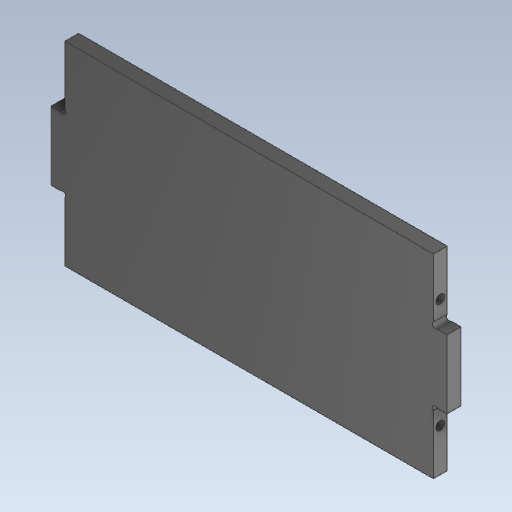
# Autodesk Inventor part: Cockpit_back_frame
Saved by Autodesk Inventor 2020.4 (Build 244396000, 396)
## iProperties
Created: 2022-01-20
Part Number: Cockpit_back_frame
Material: アセタール樹脂、黒
Document SubType Name: Modeling
Designer: Masato Kubotera
Density: 1.425 g/cm^3
Appearance: 滑らか - 黒
Author: Masato Kubotera
Autodesk Inventor part; units mm, degrees
ref_plane "XZ Plane" through (0, 0, 0) normal (0, 1, 0) x (-1, 0, 0)
ref_plane "XY Plane" through (0, 0, 0) normal (0, 0, 1) x (1, 0, 0)
derived "Cockpit_side_frame.ipt"
sketch "スケッチ1" plane through (0, 0, 0) normal (0, 1, 0) x (-1, 0, 0)
  line L0 (-60, 36.75) -> (60, 36.75) construction
  line L1 (60, 36.75) -> (60, -36.75) construction
  line L2 (60, -36.75) -> (-60, -36.75) construction
  line L3 (-60, -36.75) -> (-60, 36.75) construction
  line L4 (-60, 36.75) -> (60, -36.75) construction
  line L5 (60, 36.75) -> (-60, -36.75) construction
  line L6 (-52.5, 6.75) -> (52.5, 6.75) construction
  line L7 (52.5, 6.75) -> (52.5, 1.75) construction
  line L8 (52.5, 1.75) -> (-52.5, 1.75) construction
  line L9 (-52.5, 1.75) -> (-52.5, 6.75) construction
  line L10 (-52.5, 6.75) -> (52.5, 1.75) construction
  line L11 (52.5, 6.75) -> (-52.5, 1.75) construction
  line L12 (0, 36.75) -> (0, -36.75) construction
  line L13 (-57.5, 34.25) -> (-52.5, 34.25) construction
  line L14 (-52.5, 34.25) -> (-52.5, -34.25) construction
  line L15 (-52.5, -34.25) -> (-57.5, -34.25) construction
  line L16 (-57.5, -34.25) -> (-57.5, 34.25) construction
  line L17 (-57.5, 34.25) -> (-52.5, -34.25) construction
  line L18 (-52.5, 34.25) -> (-57.5, -34.25) construction
  line L19 (-55, 36.75) -> (-60, 31.75)
  line L20 (-60, 0) -> (60, 0) construction
  line L21 (-46.5, 41.75) -> (32.5, 41.75) construction
  line L22 (32.5, 41.75) -> (32.5, 11.75) construction
  line L23 (32.5, 11.75) -> (-46.5, 11.75) construction
  line L24 (-46.5, 11.75) -> (-46.5, 41.75) construction
  line L25 (-46.5, 41.75) -> (32.5, 11.75) construction
  line L26 (32.5, 41.75) -> (-46.5, 11.75) construction
  line L27 (-55, -36.75) -> (-60, -31.75)
  line L28 (-60, 31.75) -> (-60, -31.75)
  line L29 (55, -36.75) -> (60, -31.75)
  line L30 (-52.5, -29.25) -> (52.5, -29.25) construction
  line L31 (52.5, -29.25) -> (52.5, -34.25) construction
  line L32 (52.5, -34.25) -> (-52.5, -34.25) construction
  line L33 (-52.5, -34.25) -> (-52.5, -29.25) construction
  line L34 (-52.5, -29.25) -> (52.5, -34.25) construction
  line L35 (52.5, -29.25) -> (-52.5, -34.25) construction
  line L36 (-25, -29.25) -> (-25, -34.25) construction
  line L37 (-55, -34.25) -> (-55, 34.25) construction
  line L38 (-57.5, 12.5) -> (-52.5, 12.5) construction
  line L39 (-57.55, 12.55) -> (-52.45, 12.55)
  line L40 (-52.45, 12.55) -> (-52.45, -12.55)
  line L41 (-52.45, -12.55) -> (-57.55, -12.55)
  line L42 (-57.55, -12.55) -> (-57.55, 12.55)
  line L43 (-57.55, 12.55) -> (-52.45, -12.55) construction
  line L44 (-52.45, 12.55) -> (-57.55, -12.55) construction
  arc A0 (-52.45, 11.0651) -> (-53.9349, 12.55) centre (-53.1925, 11.8075) ccw
  circle A1 centre (-55, 20) radius 1.6
  circle A2 centre (-55, -20) radius 1.6
  arc A3 (-53.9349, -12.55) -> (-52.45, -11.0651) centre (-53.1925, -11.8075) ccw
  line L45 (-57.5, -12.5) -> (-52.5, -12.5) construction
  arc A4 (-56.0651, 12.55) -> (-57.55, 11.0651) centre (-56.8075, 11.8075) ccw
  arc A5 (-57.55, -11.0651) -> (-56.0651, -12.55) centre (-56.8075, -11.8075) ccw
  line L46 (-52.5, -31.75) -> (52.5, -31.75) construction
  line L47 (-25.05, -34.3) -> (-25.05, -29.2)
  line L48 (-25.05, -29.2) -> (25.05, -29.2)
  circle A6 centre (-32.5, -31.75) radius 1.6
  circle A7 centre (32.5, -31.75) radius 1.6
  line L49 (25, -29.25) -> (25, -34.25) construction
  line L50 (52.5, 36.75) -> (57.5, 36.75) construction
  line L51 (57.5, 36.75) -> (57.5, -34.25) construction
  line L52 (57.5, -34.25) -> (52.5, -34.25) construction
  line L53 (52.5, -34.25) -> (52.5, 36.75) construction
  line L54 (52.5, 36.75) -> (57.5, -34.25) construction
  line L55 (57.5, 36.75) -> (52.5, -34.25) construction
  line L56 (52.5, 1.25) -> (57.5, 1.25) construction
  line L57 (52.5, -11.25) -> (57.5, -11.25) construction
  line L58 (55, -34.25) -> (55, 36.75) construction
  circle A8 centre (55, -18.75) radius 1.6
  line L59 (60, -11.3) -> (52.45, -11.3)
  line L60 (52.45, -11.3) -> (52.45, 13.8)
  arc A9 (52.45, -9.8151) -> (53.9349, -11.3) centre (53.1925, -10.5575) ccw
  line L61 (60, 13.8) -> (52.45, 13.8)
  arc A10 (53.9349, 13.8) -> (52.45, 12.3151) centre (53.1925, 13.0575) ccw
  line L62 (52.5, 13.75) -> (57.5, 13.75) construction
  circle A11 centre (55, 21.25) radius 1.6
  arc A12 (-23.5651, -29.2) -> (-25.05, -30.6849) centre (-24.3075, -29.9425) ccw
  arc A13 (25.05, -30.6849) -> (23.5651, -29.2) centre (24.3075, -29.9425) ccw
  circle A14 centre (-55, 20) radius 3
  circle A15 centre (-32.5, -31.75) radius 3
  circle A16 centre (-55, -20) radius 3
  circle A17 centre (32.5, -31.75) radius 3
  line L63 (25.05, -34.3) -> (25.05, -29.2)
  line L64 (25.05, 6.8) -> (-25.05, 6.8)
  line L65 (-25.05, 6.8) -> (-25.05, 1.7)
  line L66 (-25.05, 1.7) -> (25.05, 1.7)
  line L67 (25.05, 1.7) -> (25.05, 6.8)
  line L68 (25.05, 6.8) -> (-25.05, 1.7) construction
  line L69 (-25.05, 6.8) -> (25.05, 1.7) construction
  line L70 (-25, 6.75) -> (-25, 1.75) construction
  arc A18 (-23.5651, 6.8) -> (-25.05, 5.3151) centre (-24.3075, 6.0575) ccw
  line L71 (52.5, 4.25) -> (-52.5, 4.25) construction
  circle A19 centre (-32.5, 4.25) radius 1.6
  line L72 (25, 6.75) -> (25, 1.75) construction
  arc A20 (25.05, 5.3151) -> (23.5651, 6.8) centre (24.3075, 6.0575) ccw
  circle A21 centre (32.5, 4.25) radius 1.6
  arc A22 (-25.05, 3.1849) -> (-23.5651, 1.7) centre (-24.3075, 2.4425) ccw
  arc A23 (23.5651, 1.7) -> (25.05, 3.1849) centre (24.3075, 2.4425) ccw
  line L73 (60, 31.75) -> (60, 13.8)
  line L74 (60, -11.3) -> (60, -31.75)
  circle A24 centre (-32.5, 4.25) radius 3
  circle A25 centre (55, -18.75) radius 3
  circle A26 centre (55, 21.25) radius 3
  circle A27 centre (32.5, 4.25) radius 3
  line L75 (60, 31.75) -> (60, 39.25)
  line L76 (21, 36.75) -> (-55, 36.75)
  line L77 (60, 39.25) -> (57.5, 41.75)
  line L78 (57.5, 41.75) -> (50, 41.75)
  line L79 (50, 41.75) -> (50, 36.75)
  line L80 (50, 36.75) -> (40.5, 36.75)
  line L81 (40.5, 36.75) -> (40.5, 41.75)
  line L82 (40.5, 41.75) -> (30.5, 41.75)
  line L83 (30.5, 41.75) -> (30.5, 36.75)
  line L84 (30.5, 36.75) -> (21, 36.75)
  line L85 (21, 36.75) -> (21, 36.75)
  circle A28 centre (-45, 4.25) radius 1.75
  line L86 (35.5, 41.75) -> (35.5, 36.75) construction
  line L87 (37.9, -8.6) -> (47.1, -8.6) construction
  line L88 (47.1, -8.6) -> (47.1, -22.4) construction
  line L89 (47.1, -22.4) -> (37.9, -22.4) construction
  line L90 (37.9, -22.4) -> (37.9, -8.6) construction
  line L91 (37.9, -8.6) -> (47.1, -22.4) construction
  line L92 (47.1, -8.6) -> (37.9, -22.4) construction
  line L93 (37.2, -7.95) -> (47.8, -7.95) construction
  line L94 (47.8, -7.95) -> (47.8, -23.05) construction
  line L95 (47.8, -23.05) -> (37.2, -23.05) construction
  line L96 (37.2, -23.05) -> (37.2, -7.95) construction
  line L97 (37.2, -7.95) -> (47.8, -23.05) construction
  line L98 (47.8, -7.95) -> (37.2, -23.05) construction
  line L99 (42.5, -7.95) -> (42.5, -23.05) construction
  line L100 (47.8, -15.5) -> (37.2, -15.5) construction
  line L101 (38.6349, -7.9) -> (46.3651, -7.9)
  line L102 (37.15, -9.3849) -> (37.15, -21.6151)
  line L103 (39.3349, -8.55) -> (45.6651, -8.55)
  line L104 (37.85, -10.0349) -> (37.85, -20.9651)
  arc A29 (38.6349, -7.9) -> (37.15, -9.3849) centre (37.8925, -8.6425) ccw
  arc A30 (39.3349, -8.55) -> (37.85, -10.0349) centre (38.5925, -9.2925) ccw
  arc A31 (47.85, -9.3849) -> (46.3651, -7.9) centre (47.1075, -8.6425) ccw
  arc A32 (47.15, -10.0349) -> (45.6651, -8.55) centre (46.4075, -9.2925) ccw
  line L105 (38.6349, -23.1) -> (46.3651, -23.1)
  line L106 (39.3349, -22.45) -> (45.6651, -22.45)
  arc A33 (37.85, -20.9651) -> (39.3349, -22.45) centre (38.5925, -21.7075) ccw
  arc A34 (37.15, -21.6151) -> (38.6349, -23.1) centre (37.8925, -22.3575) ccw
  arc A35 (46.3651, -23.1) -> (47.85, -21.6151) centre (47.1075, -22.3575) ccw
  arc A36 (45.6651, -22.45) -> (47.15, -20.9651) centre (46.4075, -21.7075) ccw
  line L107 (47.15, -10.0349) -> (47.15, -20.9651)
  line L108 (47.85, -9.3849) -> (47.85, -21.6151)
  line L109 (-45.5, -4.25) -> (10.5, -4.25)
  line L110 (12.5, -6.25) -> (12.5, -22.25)
  line L111 (10.5, -24.25) -> (-45.5, -24.25)
  line L112 (-47.5, -22.25) -> (-47.5, -6.25)
  line L113 (-47.5, -4.25) -> (12.5, -24.25) construction
  line L114 (12.5, -4.25) -> (-47.5, -24.25) construction
  arc A37 (-45.5, -4.25) -> (-47.5, -6.25) centre (-45.5, -6.25) ccw
  arc A38 (-47.5, -22.25) -> (-45.5, -24.25) centre (-45.5, -22.25) ccw
  arc A39 (10.5, -24.25) -> (12.5, -22.25) centre (10.5, -22.25) ccw
  arc A40 (12.5, -6.25) -> (10.5, -4.25) centre (10.5, -6.25) ccw
  line L115 (26.5, 36.75) -> (26.5, 32.75) construction
  line L116 (24.5, 32.75) -> (28.5, 32.75) construction
  line L117 (28.5, 32.75) -> (28.5, 36.75) construction
  line L118 (24.5, 32.75) -> (24.5, 36.75) construction
  line L119 (42.5, 32.75) -> (42.5, 36.75) construction
  line L120 (44.5, 36.75) -> (44.5, 32.75) construction
  line L121 (46.5, 32.75) -> (42.5, 32.75) construction
  line L122 (46.5, 32.75) -> (46.5, 36.75) construction
  arc A41 (48.5151, 36.75) -> (50, 38.2349) centre (49.2575, 37.4925) ccw
  arc A42 (29.0151, 36.75) -> (30.5, 38.2349) centre (29.7575, 37.4925) ccw
  arc A43 (40.5, 38.2349) -> (41.9849, 36.75) centre (41.2425, 37.4925) ccw
  line L123 (30.5, 36.75) -> (40.5, 36.75)
  line L124 (60, -36.75) -> (60, -79.25)
  line L125 (60, -79.25) -> (14, -79.25)
  line L126 (9, -74.25) -> (9, -36.75)
  arc A44 (-25.05, -32.8151) -> (-23.5651, -34.3) centre (-24.3075, -33.5575) ccw
  arc A45 (23.5651, -34.3) -> (25.05, -32.8151) centre (24.3075, -33.5575) ccw
  line L127 (60, -36.75) -> (60, -31.75)
  line L128 (-25.05, -34.3) -> (25.05, -34.3)
  line L129 (-55, -36.75) -> (9, -36.75)
  line L130 (16.5, -48.75) -> (50.5, -48.75) construction
  line L131 (50.5, -48.75) -> (50.5, -71.75) construction
  line L132 (50.5, -71.75) -> (16.5, -71.75) construction
  line L133 (16.5, -71.75) -> (16.5, -48.75) construction
  line L134 (16.5, -48.75) -> (50.5, -71.75) construction
  line L135 (50.5, -48.75) -> (16.5, -71.75) construction
  line L136 (14, -45.5) -> (16.5, -45.5) construction
  line L137 (16.5, -45.5) -> (16.5, -60.5) construction
  line L138 (16.5, -60.5) -> (14, -60.5) construction
  line L139 (14, -60.5) -> (14, -45.5) construction
  line L140 (14, -45.5) -> (16.5, -60.5) construction
  line L141 (16.5, -45.5) -> (14, -60.5) construction
  line L142 (13.95, -45.45) -> (16.55, -45.45)
  line L143 (16.55, -45.45) -> (16.55, -60.55)
  line L144 (16.55, -60.55) -> (13.95, -60.55)
  line L145 (13.95, -60.55) -> (13.95, -45.45)
  line L146 (13.95, -45.45) -> (16.55, -60.55) construction
  line L147 (16.55, -45.45) -> (13.95, -60.55) construction
  line L148 (15.25, -45.5) -> (15.25, -60.5) construction
  line L149 (14, -53) -> (16.5, -53) construction
  arc A46 (15.4349, -45.45) -> (13.95, -46.9349) centre (14.6925, -46.1925) ccw
  arc A47 (16.55, -47.55) -> (16.55, -45.45) centre (16.55, -46.5) ccw
  arc A48 (13.95, -59.0651) -> (15.4349, -60.55) centre (14.6925, -59.8075) ccw
  arc A49 (16.55, -60.55) -> (16.55, -58.45) centre (16.55, -59.5) ccw
  line L150 (11.5, -34.25) -> (16.5, -34.25) construction
  line L151 (16.5, -34.25) -> (16.5, -71.75) construction
  line L152 (16.5, -71.75) -> (11.5, -71.75) construction
  line L153 (11.5, -71.75) -> (11.5, -34.25) construction
  line L154 (11.5, -34.25) -> (16.5, -71.75) construction
  line L155 (16.5, -34.25) -> (11.5, -71.75) construction
  circle A50 centre (14, -39.5) radius 1.6
  line L156 (14, -34.25) -> (14, -71.75) construction
  circle A51 centre (14, -66.5) radius 1.6
  line L157 (14, -79.25) -> (9, -74.25)
  circle A52 centre (14, -39.5) radius 3
  circle A53 centre (14, -66.5) radius 3
  line L158 (11.5, -71.75) -> (50, -71.75) construction
  line L159 (50, -71.75) -> (50, -76.75) construction
  line L160 (50, -76.75) -> (11.5, -76.75) construction
  line L161 (11.5, -76.75) -> (11.5, -71.75) construction
  line L162 (11.5, -71.75) -> (50, -76.75) construction
  line L163 (50, -71.75) -> (11.5, -76.75) construction
  line L164 (30.75, -76.75) -> (30.75, -71.75) construction
  line L165 (11.5, -74.25) -> (50, -74.25) construction
  line L166 (25.75, -71.75) -> (35.75, -71.75) construction
  line L167 (35.75, -71.75) -> (35.75, -74.25) construction
  line L168 (35.75, -74.25) -> (25.75, -74.25) construction
  line L169 (25.75, -74.25) -> (25.75, -71.75) construction
  line L170 (25.75, -71.75) -> (35.75, -74.25) construction
  line L171 (35.75, -71.75) -> (25.75, -74.25) construction
  line L172 (25.7, -71.7) -> (35.8, -71.7)
  line L173 (35.8, -71.7) -> (35.8, -74.3)
  line L174 (35.8, -74.3) -> (25.7, -74.3)
  line L175 (25.7, -74.3) -> (25.7, -71.7)
  line L176 (25.7, -71.7) -> (35.8, -74.3) construction
  line L177 (35.8, -71.7) -> (25.7, -74.3) construction
  arc A54 (25.7, -72.8151) -> (27.1849, -74.3) centre (26.4425, -73.5575) ccw
  arc A55 (27.8, -71.7) -> (25.7, -71.7) centre (26.75, -71.7) ccw
  arc A56 (34.3151, -74.3) -> (35.8, -72.8151) centre (35.0575, -73.5575) ccw
  arc A57 (35.8, -71.7) -> (33.7, -71.7) centre (34.75, -71.7) ccw
  circle A58 centre (42.75, -74.25) radius 1.6
  circle A59 centre (42.75, -74.25) radius 3
  point P0 (0, 0)
  point P1 (0, 4.25)
  point P2 (-55, 0)
  point P3 (-55, 0)
  point P4 (-7, 26.75)
  point P5 (0, -31.75)
  point P6 (-25.05, -34.25)
  point P7 (25.05, -34.25)
  point P8 (0, 4.25)
  point P9 (42.5, -15.5)
  point P10 (37.15, -7.9)
  point P11 (37.85, -8.55)
  point P12 (-17.5, -14.25)
  point P13 (9, -79.25)
  point P14 (33.5, -60.25)
  point P15 (15.25, -53)
  point P16 (30.75, -74.25)
  point P17 (30.75, -73)
  dimension "d1" = 52.5
  dimension "d2" = 71
  dimension "d3" = 40
  dimension "d5" = 25
  measures "d1" horizontal distance of L7.end point (0, 0)
  measures "d2" distance of L50.end L51.end
  measures "d3" distance of A8.centre A11.centre
  measures "d5" distance of L57.end L62.end
ref_plane "作業平面1" through (-52.5, 0, 0) normal (1, 0, 0) x (0, 1, 0)
sketch "スケッチ2" plane through (-52.5, 0, 0) normal (1, 0, 0) x (0, 1, 0)
  line L0 (-134.5, 36.75) -> (0, 36.75)
  line L1 (0, 36.75) -> (0, -34.25) construction
  line L2 (0, -34.25) -> (-134.5, -34.25)
  line L3 (-134.5, -34.25) -> (-134.5, 36.75) construction
  line L4 (-134.5, 36.75) -> (0, -34.25) construction
  line L5 (0, 36.75) -> (-134.5, -34.25) construction
  line L6 (-67.25, 36.75) -> (-67.25, -34.25) construction
  line L7 (0, 13.75) -> (5, 13.75)
  line L8 (5, 13.75) -> (5, -11.25)
  arc A0 (0, 15.2349) -> (1.4849, 13.75) centre (0.7425, 14.4925) ccw
  line L9 (0, 1.25) -> (-134.5, 1.25) construction
  line L10 (0, -11.25) -> (5, -11.25)
  arc A1 (1.4849, -11.25) -> (0, -12.7349) centre (0.7425, -11.9925) ccw
  line L11 (0, 36.75) -> (0, 15.2349)
  line L12 (0, -12.7349) -> (0, -34.25)
  line L13 (-134.5, 13.75) -> (-139.5, 13.75)
  line L14 (-139.5, 13.75) -> (-139.5, -11.25)
  arc A2 (-135.9849, 13.75) -> (-134.5, 15.2349) centre (-135.2425, 14.4925) ccw
  line L15 (-134.5, -11.25) -> (-139.5, -11.25)
  arc A3 (-134.5, -12.7349) -> (-135.9849, -11.25) centre (-135.2425, -11.9925) ccw
  line L16 (-134.5, -12.7349) -> (-134.5, -34.25)
  line L17 (-134.5, 36.75) -> (-134.5, 15.2349)
  point P0 (-67.25, 1.25)
  point P1 (5, 1.25)
  dimension "d7" = 134.5
  dimension "d8" = 71
  dimension "d9" = 1.05
  dimension "d10" = 5
  dimension "d11" = 25
  constraints: 37 end point, 14 symmetric about line, 9 point on circle, 7 midpoint, 7 point on line, 4 centre point, 3 perpendicular, 2 horizontal, 2 parallel, 1 coincident, 1 collinear, 3 other
  measures "d7" distance of L0.start L0.end
  measures "d8" distance of L0.end L1.end
  measures "d9" radius of A0
  measures "d10" distance of L7.start L7.end
  measures "d11" distance of L7.end L8.end
extrude "押し出し1" add sketch "スケッチ2" against normal blind 5 contours L0 L11 A0 L7 L8 L10 A1 L12 L2 L16 A3 L15 L14 L13 A2 L17
hole "穴1" at (-55, 0, 21.25) at (-55, 0, -18.75) direction (0, -1, 0) diameter 3.242 depth 11.8 tip angle 118 thread size "M4x0.7" class "6H" standard "ISO Metric profile"
equation "\"d8\" = d2"
equation "\"d11\" = d5"
equation "\"d6\" = -d1"
